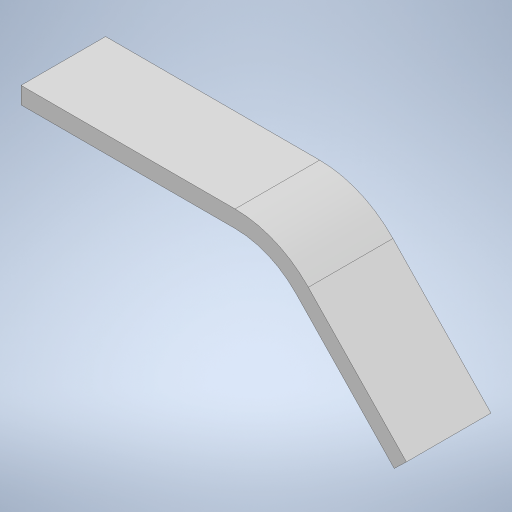
# Autodesk Inventor part: 1p5 sensor for show
Saved by Autodesk Inventor 2024.2 (Build 282272000, 272)
## iProperties
Created: 2024-11-21
Part Number: 1p5 sensor for show
Material: Generic
Document SubType Name: Modeling
Designer: Tom
Density: 1 g/cm^3
Appearance: Default
Author: Tom
Autodesk Inventor part; units mm, degrees
ref_plane "YZ Plane" through (0, 0, 0) normal (1, 0, 0) x (0, 1, 0)
ref_plane "XZ Plane" through (0, 0, 0) normal (0, 1, 0) x (-1, 0, 0)
ref_plane "XY Plane" through (0, 0, 0) normal (0, 0, 1) x (1, 0, 0)
sketch "Sketch1" plane through (0, 0, 0) normal (0, 0, 1) x (1, 0, 0)
  line L0 (0, 0) -> (16.0718, 0)
  line L1 (21.1119, -2.149) -> (24.2127, -5.3806)
  arc A0 (21.1119, -2.149) -> (16.0718, 0) centre (16.0718, -6.985) ccw
  line L2 (24.2127, -5.3806) -> (28.4753, -9.8231)
  point P0 (19.05, 0)
  dimension "d0" = 19.05
  dimension "d1" = 6.985
  constraints: 6 end point, 2 point on circle, 2 point on line, 2 tangent, 1 centre point, 1 horizontal
  measures "d0" distance of L0.start point (19.05, 0)
  measures "d1" radius of A0
sketch "Sketch2" plane through (0, 0, 0) normal (1, 0, 0) x (0, 1, 0)
  line L0 (0.635, -3.175) -> (-0.635, -3.175)
  line L1 (-0.635, -3.175) -> (-0.635, 3.175)
  line L2 (-0.635, 3.175) -> (0.635, 3.175)
  line L3 (0.635, 3.175) -> (0.635, -3.175)
  line L4 (0.635, -3.175) -> (-0.635, 3.175) construction
  line L5 (-0.635, -3.175) -> (0.635, 3.175) construction
  point P0 (0, 0)
  dimension "d2" = 1.27
  dimension "d3" = 6.35
  constraints: 12 end point, 2 midpoint, 2 parallel, 1 horizontal, 1 perpendicular
  measures "d2" distance of L1.end L2.end
  measures "d3" distance of L2.end L0.start
sweep "Sweep1" add profiles "Sketch2" path "Sketch1"
body "Solid1"
